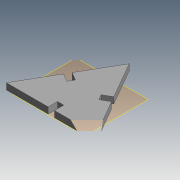
# Autodesk Inventor part: Lower PlatformV
Saved by Autodesk Inventor 2014 SP1 (Build 180222100, 222)
## iProperties
Created: 2014-04-09
Part Number: Lower PlatformV
Material: Generic
Document SubType Name: Modeling
Designer: tom
Density: 1 g/cm^3
Appearance: Default
Author: tom
Autodesk Inventor part; units mm, degrees
ref_plane "YZ Plane" through (0, 0, 0) normal (1, 0, 0) x (0, 1, 0)
ref_plane "XZ Plane" through (0, 0, 0) normal (0, 1, 0) x (-1, 0, 0)
ref_plane "XY Plane" through (0, 0, 0) normal (0, 0, 1) x (1, 0, 0)
ref_plane "Work Plane1" through (64.8465, 16.6938, -6.1656) normal (0, 1, 0) x (1, 0, 0)
sketch "Sketch1" plane through (64.8465, 16.6938, -6.1656) normal (0, 1, 0) x (1, 0, 0)
  line L0 (1.7321, 1) -> (27.6872, 15.9852) construction
  line L1 (13.1559, 10.8634) -> (20.3785, 15.0334)
  line L2 (15.9859, 5.9616) -> (23.2085, 10.1316)
  line L3 (13.1559, 10.8634) -> (15.9859, 5.9616)
  circle A0 centre (1.7321, 1) radius 20 construction
  circle A1 centre (19.0526, 11) radius 5.175 construction
  line L4 (1.7321, 47.33) -> (20.3785, 15.0334)
  line L5 (23.2085, 10.1316) -> (41.855, -22.165)
  line L6 (-12.5218, 5.9616) -> (-19.7444, 10.1316)
  line L7 (-9.6918, 10.8634) -> (-16.9144, 15.0334)
  line L8 (-12.5218, 5.9616) -> (-9.6918, 10.8634)
  line L9 (4.5621, -13.825) -> (4.5621, -22.165)
  line L10 (-1.0979, -13.825) -> (-1.0979, -22.165)
  line L11 (4.5621, -13.825) -> (-1.0979, -13.825)
  line L12 (1.7321, 47.33) -> (-16.9144, 15.0334)
  line L13 (-19.7444, 10.1316) -> (-38.3909, -22.165)
  line L14 (-38.3909, -22.165) -> (-1.0979, -22.165)
  line L15 (4.5621, -22.165) -> (41.855, -22.165)
  dimension "d34" = 40
  dimension "d35" = 10.35
  dimension "d38" = 360
  constraints: 32 end point, 3 parallel, 1 centre point, 1 coincident, 1 point on line, 25 other
  measures "d35" diameter of A1
extrude "Extrusion2" add sketch "Sketch1" along normal blind 5.66
body "Solid2"
